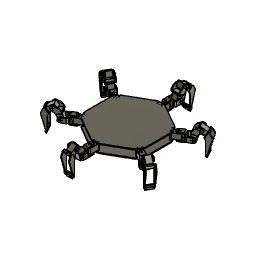
Final Iteration for VREP (Autodesk Fusion 360 design; units mm, degrees)
Autodesk Fusion 360 part; units mm, degrees
(part 1 of 2)
sketch "Sketch1" plane through (0, 0, 0) normal (0, 0, 1) x (1, 0, 0)
  line L0 (-115.223, -83.8445) -> (-15, -141.7083)
  circle A0 centre (-8, 136.7083) radius 1
  circle A1 centre (122.3929, -61.426) radius 1
  line L1 (0, 0) -> (-182.8649, -105.5771) construction
  circle A2 centre (0, 0) radius 142.5 construction
  circle A3 centre (-114.3929, -75.2824) radius 1
  line L2 (0, 0) -> (-200, 0) construction
  line L3 (-15, 141.7083) -> (15, 141.7083)
  line L4 (115.223, 83.8445) -> (15, 141.7083)
  line L5 (-15, -141.7083) -> (15, -141.7083)
  circle A4 centre (114.3929, 75.2824) radius 1
  circle A5 centre (122.3929, 61.426) radius 1
  circle A6 centre (-122.3929, -61.426) radius 1
  line L6 (0, 0) -> (0, 70) construction
  line L7 (-15, 141.7083) -> (-115.223, 83.8445)
  line L8 (-130.223, -57.8638) -> (-115.223, -83.8445)
  circle A7 centre (114.3929, -75.2824) radius 1
  line L9 (-130.223, 57.8638) -> (-130.223, -57.8638)
  line L10 (15, -141.7083) -> (115.223, -83.8445)
  line L11 (130.223, -57.8638) -> (130.223, 57.8638)
  line L12 (130.223, 57.8638) -> (115.223, 83.8445)
  circle A8 centre (-8, -136.7083) radius 1
  circle A9 centre (8, -136.7083) radius 1
  circle A10 centre (-114.3929, 75.2824) radius 1
  line L13 (130.223, -57.8638) -> (115.223, -83.8445)
  circle A11 centre (-122.3929, 61.426) radius 1
  line L14 (-130.223, 57.8638) -> (-115.223, 83.8445)
  line L15 (-128.4918, -62.4457) -> (-84.3692, -138.8683) construction
  circle A12 centre (8, 136.7083) radius 1
  dimension "d1" = 285
  dimension "d2" = 30
  dimension "d3" = 30
  dimension "d4" = 2
  dimension "d5" = 5
  dimension "d6" = 8
  dimension "d7" = 2
  dimension "d8" = 16
  dimension "d9" = 30
  dimension "d10" = 2
  dimension "d11" = 30
  dimension "d12" = 15
  dimension "d13" = 5
  dimension "d14" = 8
  dimension "d15" = 5
  constraint coincident L1.start A2.centre
  constraint coincident L0.end A2
  constraint coincident L5.end A2
  constraint horizontal L5
  constraint coincident L3.start A2
  constraint coincident L3.end A2
  constraint horizontal L3
  constraint parallel L2 L3
  constraint perpendicular L1 L15
  constraint tangent A2 L15
  constraint coincident L8.start A2
  constraint coincident L0.start A2
  constraint symmetric L1 A3 A6
  constraint symmetric A3 L2 A10
  constraint symmetric L8.start L9.start L2
  constraint symmetric L7.end L0.start L2
  constraint symmetric L2 A6 A11
  constraint perpendicular L2 L6
  constraint symmetric A3 L6 A7
  constraint symmetric L8.start L11.start L6
  constraint symmetric L10.end L0.start L6
  constraint symmetric A1 A6 L6
  constraint symmetric A5 L6 A11
  constraint symmetric A4 L6 A10
  constraint symmetric L11.end L9.start L6
  constraint symmetric L7.end L4.start L6
  constraint symmetric L2 A9 A12
  constraint symmetric A0 L2 A8
  measures "d1" diameter of A2
  measures "d2" distance of L5.end L0.end
  measures "d3" distance of L3.start L3.end
  measures "d4" diameter of A12
  measures "d5" distance of A12.centre L3
  measures "d6" horizontal distance of L1.start A12.centre
  measures "d7" diameter of A0
  measures "d8" horizontal distance of A12.centre A0.centre
  measures "d9" angle of L1 L2
  measures "d10" diameter of A3
  measures "d11" distance of L8.start L0.start
  measures "d12" distance of L0.start L1
  measures "d13" distance of A3.centre L8
  measures "d14" distance of A3.centre L1
  measures "d15" distance of A0.centre L3
extrude "Extrude1" add sketch "Sketch1" along normal blind 3.5 makes body 1
sketch "Sketch2" plane through (0, 0, 3.5) normal (0, 0, 1) x (-1, 0, 0)
  circle A0 centre (8, -136.7083) radius 1
  circle A1 centre (122.3929, 61.426) radius 1
  circle A2 centre (8, 136.7083) radius 1
  circle A3 centre (114.3929, -75.2824) radius 1
  circle A4 centre (-114.3929, 75.2824) radius 1
  circle A5 centre (-122.3929, 61.426) radius 1
  circle A6 centre (114.3929, 75.2824) radius 1
  circle A7 centre (-114.3929, -75.2824) radius 1
  circle A8 centre (-122.3929, -61.426) radius 1
  circle A9 centre (122.3929, -61.426) radius 1
  circle A10 centre (-8, -136.7083) radius 1
  circle A11 centre (-8, 136.7083) radius 1
  line L0 (130.223, 57.8638) -> (115.223, 83.8445)
  line L1 (115.223, 83.8445) -> (15, 141.7083)
  line L2 (15, 141.7083) -> (-15, 141.7083)
  line L3 (-15, 141.7083) -> (-115.223, 83.8445)
  line L4 (-115.223, 83.8445) -> (-130.223, 57.8638)
  line L5 (-130.223, 57.8638) -> (-130.223, -57.8638)
  line L6 (-130.223, -57.8638) -> (-115.223, -83.8445)
  line L7 (-115.223, -83.8445) -> (-15, -141.7083)
  line L8 (-15, -141.7083) -> (15, -141.7083)
  line L9 (15, -141.7083) -> (115.223, -83.8445)
  line L10 (115.223, -83.8445) -> (130.223, -57.8638)
  line L11 (130.223, -57.8638) -> (130.223, 57.8638)
  circle A12 centre (-122.3929, 61.426) radius 1
  circle A13 centre (-114.3929, 75.2824) radius 1
  circle A14 centre (-8, 136.7083) radius 1
  circle A15 centre (8, 136.7083) radius 1
  circle A16 centre (114.3929, 75.2824) radius 1
  circle A17 centre (122.3929, 61.426) radius 1
  line L12 (-115.223, 83.8445) -> (-130.223, 57.8638)
  line L13 (15, 141.7083) -> (-15, 141.7083)
  line L14 (130.223, 57.8638) -> (115.223, 83.8445)
  line L15 (115.223, 83.8445) -> (130.223, 57.8638)
  line L16 (-114.3929, 75.2824) -> (-110.0628, 72.7824) construction
  line L17 (-110.0628, 72.7824) -> (-108.5628, 75.3804) construction
  line L18 (-108.5628, 75.3804) -> (-112.8929, 77.8804)
  line L19 (-108.5628, 75.3804) -> (-108.6561, 75.2188)
  line L20 (-108.5628, 75.3804) -> (-119.5628, 56.3279)
  line L21 (-119.5628, 56.3279) -> (-123.8929, 58.8279)
  arc A18 (-112.8929, 77.8804) -> (-115.8929, 72.6843) centre (-114.3929, 75.2824) ccw
  arc A19 (-120.8929, 64.024) -> (-123.8929, 58.8279) centre (-122.3929, 61.426) ccw
  line L22 (-120.8929, 64.024) -> (-115.8929, 72.6843)
  line L23 (-108.5628, -75.3804) -> (-112.8929, -77.8804)
  arc A20 (-115.8929, -72.6843) -> (-112.8929, -77.8804) centre (-114.3929, -75.2824) ccw
  line L24 (-115.8929, -72.6843) -> (-120.8929, -64.024)
  arc A21 (-123.8929, -58.8279) -> (-120.8929, -64.024) centre (-122.3929, -61.426) ccw
  line L25 (-119.5628, -56.3279) -> (-123.8929, -58.8279)
  line L26 (-119.5628, -56.3279) -> (-108.5628, -75.3804)
  line L27 (11, -131.7083) -> (11, -136.7083)
  arc A22 (5, -136.7083) -> (11, -136.7083) centre (8, -136.7083) ccw
  line L28 (5, -136.7083) -> (-5, -136.7083)
  arc A23 (-11, -136.7083) -> (-5, -136.7083) centre (-8, -136.7083) ccw
  line L29 (-11, -131.7083) -> (-11, -136.7083)
  line L30 (-11, -131.7083) -> (11, -131.7083)
  line L31 (119.5628, -56.3279) -> (123.8929, -58.8279)
  arc A24 (120.8929, -64.024) -> (123.8929, -58.8279) centre (122.3929, -61.426) ccw
  line L32 (120.8929, -64.024) -> (115.8929, -72.6843)
  arc A25 (112.8929, -77.8804) -> (115.8929, -72.6843) centre (114.3929, -75.2824) ccw
  line L33 (108.5628, -75.3804) -> (112.8929, -77.8804)
  line L34 (108.5628, -75.3804) -> (119.5628, -56.3279)
  line L35 (108.5628, 75.3804) -> (112.8929, 77.8804)
  arc A26 (115.8929, 72.6843) -> (112.8929, 77.8804) centre (114.3929, 75.2824) ccw
  line L36 (115.8929, 72.6843) -> (120.8929, 64.024)
  arc A27 (123.8929, 58.8279) -> (120.8929, 64.024) centre (122.3929, 61.426) ccw
  line L37 (119.5628, 56.3279) -> (123.8929, 58.8279)
  line L38 (119.5628, 56.3279) -> (108.5628, 75.3804)
  line L39 (-11, 131.7083) -> (-11, 136.7083)
  arc A28 (-5, 136.7083) -> (-11, 136.7083) centre (-8, 136.7083) ccw
  line L40 (-5, 136.7083) -> (5, 136.7083)
  arc A29 (11, 136.7083) -> (5, 136.7083) centre (8, 136.7083) ccw
  line L41 (11, 131.7083) -> (11, 136.7083)
  line L42 (11, 131.7083) -> (-11, 131.7083)
  dimension "d22" = 6
  dimension "d23" = 6
  dimension "d24" = 5
  dimension "d25" = 90
  dimension "d27" = 22
  dimension "d29" = 360
  constraint concentric A12 A19
  constraint concentric A4 A18
  constraint coincident A4.centre A13.centre
  constraint perpendicular L12 L16
  constraint perpendicular L16 L17
  constraint perpendicular L12 L18
  constraint tangent L18 A18
  constraint coincident L17 L19.end
  constraint perpendicular L18 L20
  constraint perpendicular L20 L21
  measures "d22" diameter of A19
  measures "d23" diameter of A18
  measures "d24" distance of A4.centre L16.end
  measures "d25" angle of L12 L16
  measures "d27" distance of L17.end L20.end
extrude "Extrude2" add sketch "Sketch2" along normal blind 3.5 contours L18 L19 L20 L21 A18 A19 L22 | L23 A20 L24 A21 L25 L26 | L27 A22 L28 A23 L29 L30 | L31 A24 L32 A25 L33 L34 | L35 A26 L36 A27 L37 L38 | L39 A28 L40 A29 L41 L42 bodies 1
sketch "Sketch3" plane through (0, 0, 7) normal (0, 0, 1) x (-1, 0, 0)
  circle A0 centre (122.3929, 61.426) radius 1
  circle A1 centre (114.3929, 75.2824) radius 1
  arc A2 (123.8929, 58.8279) -> (120.8929, 64.024) centre (122.3929, 61.426) ccw
  line L0 (120.8929, 64.024) -> (115.8929, 72.6843)
  arc A3 (115.8929, 72.6843) -> (112.8929, 77.8804) centre (114.3929, 75.2824) ccw
  line L1 (112.8929, 77.8804) -> (108.5628, 75.3804)
  line L2 (108.5628, 75.3804) -> (119.5628, 56.3279)
  line L3 (119.5628, 56.3279) -> (123.8929, 58.8279)
  circle A4 centre (122.3929, -61.426) radius 1
  circle A5 centre (114.3929, -75.2824) radius 1
  line L4 (114.3929, -75.2824) -> (122.3929, -61.426) construction
  line L5 (122.3929, -61.426) -> (123.3929, -59.6939) construction
  line L6 (114.3929, -75.2824) -> (113.3929, -77.0144) construction
  line L7 (114.3929, -75.2824) -> (112.6608, -74.2824) construction
  line L8 (122.3929, -61.426) -> (120.6608, -60.426) construction
  line L9 (123.3929, -59.6939) -> (151.1057, -75.6939)
  line L10 (113.3929, -77.0144) -> (141.1057, -93.0144)
  line L11 (151.1057, -75.6939) -> (141.1057, -93.0144)
  line L12 (136.3833, -67.1939) -> (132.418, -74.062) construction
  circle A6 centre (148.3736, -76.426) radius 1
  circle A7 centre (140.3736, -90.2824) radius 1
  line L13 (123.8929, -58.8279) -> (119.5628, -56.3279)
  line L14 (119.5628, -56.3279) -> (108.5628, -75.3804)
  line L15 (108.5628, -75.3804) -> (112.8929, -77.8804)
  line L16 (113.3929, -77.0144) -> (112.8929, -77.8804)
  line L17 (123.3929, -59.6939) -> (123.8929, -58.8279)
  line L18 (123.3929, 59.6939) -> (151.1057, 75.6939)
  line L19 (141.1057, 93.0144) -> (151.1057, 75.6939)
  line L20 (113.3929, 77.0144) -> (141.1057, 93.0144)
  line L21 (113.3929, 77.0144) -> (112.8929, 77.8804)
  line L22 (112.8929, 77.8804) -> (108.5628, 75.3804)
  line L23 (108.5628, 75.3804) -> (119.5628, 56.3279)
  line L24 (119.5628, 56.3279) -> (123.8929, 58.8279)
  line L25 (123.3929, 59.6939) -> (123.8929, 58.8279)
  circle A8 centre (122.3929, 61.426) radius 1
  circle A9 centre (114.3929, 75.2824) radius 1
  circle A10 centre (140.3736, 90.2824) radius 1
  circle A11 centre (148.3736, 76.426) radius 1
  line L26 (10, 136.7083) -> (10, 168.7083)
  line L27 (-10, 168.7083) -> (10, 168.7083)
  line L28 (-10, 136.7083) -> (-10, 168.7083)
  line L29 (-10, 136.7083) -> (-11, 136.7083)
  line L30 (-11, 136.7083) -> (-11, 131.7083)
  line L31 (-11, 131.7083) -> (11, 131.7083)
  line L32 (11, 131.7083) -> (11, 136.7083)
  line L33 (10, 136.7083) -> (11, 136.7083)
  circle A12 centre (8, 136.7083) radius 1
  circle A13 centre (-8, 136.7083) radius 1
  circle A14 centre (-8, 166.7083) radius 1
  circle A15 centre (8, 166.7083) radius 1
  line L34 (-113.3929, 77.0144) -> (-141.1057, 93.0144)
  line L35 (-151.1057, 75.6939) -> (-141.1057, 93.0144)
  line L36 (-123.3929, 59.6939) -> (-151.1057, 75.6939)
  line L37 (-123.3929, 59.6939) -> (-123.8929, 58.8279)
  line L38 (-123.8929, 58.8279) -> (-119.5628, 56.3279)
  line L39 (-119.5628, 56.3279) -> (-108.5628, 75.3804)
  line L40 (-108.5628, 75.3804) -> (-112.8929, 77.8804)
  line L41 (-113.3929, 77.0144) -> (-112.8929, 77.8804)
  circle A16 centre (-114.3929, 75.2824) radius 1
  circle A17 centre (-122.3929, 61.426) radius 1
  circle A18 centre (-148.3736, 76.426) radius 1
  circle A19 centre (-140.3736, 90.2824) radius 1
  line L42 (-123.3929, -59.6939) -> (-151.1057, -75.6939)
  line L43 (-141.1057, -93.0144) -> (-151.1057, -75.6939)
  line L44 (-113.3929, -77.0144) -> (-141.1057, -93.0144)
  line L45 (-113.3929, -77.0144) -> (-112.8929, -77.8804)
  line L46 (-112.8929, -77.8804) -> (-108.5628, -75.3804)
  line L47 (-108.5628, -75.3804) -> (-119.5628, -56.3279)
  line L48 (-119.5628, -56.3279) -> (-123.8929, -58.8279)
  line L49 (-123.3929, -59.6939) -> (-123.8929, -58.8279)
  circle A20 centre (-122.3929, -61.426) radius 1
  circle A21 centre (-114.3929, -75.2824) radius 1
  circle A22 centre (-140.3736, -90.2824) radius 1
  circle A23 centre (-148.3736, -76.426) radius 1
  line L50 (-10, -136.7083) -> (-10, -168.7083)
  line L51 (10, -168.7083) -> (-10, -168.7083)
  line L52 (10, -136.7083) -> (10, -168.7083)
  line L53 (10, -136.7083) -> (11, -136.7083)
  line L54 (11, -136.7083) -> (11, -131.7083)
  line L55 (11, -131.7083) -> (-11, -131.7083)
  line L56 (-11, -131.7083) -> (-11, -136.7083)
  line L57 (-10, -136.7083) -> (-11, -136.7083)
  circle A24 centre (-8, -136.7083) radius 1
  circle A25 centre (8, -136.7083) radius 1
  circle A26 centre (8, -166.7083) radius 1
  circle A27 centre (-8, -166.7083) radius 1
  point P0 (122.3929, -61.426)
  point P1 (114.3929, -75.2824)
  dimension "d32" = 2
  dimension "d33" = 2
  dimension "d34" = 2
  dimension "d35" = 2
  dimension "d39" = 32
  dimension "d43" = 360
  constraint coincident P0 A4.centre
  constraint coincident P1 A5.centre
  constraint parallel L4 L5
  constraint parallel L4 L6
  constraint perpendicular L6 L7
  constraint perpendicular L4 L8
  constraint perpendicular L5 L9
  constraint perpendicular L6 L10
  constraint perpendicular L9 L12
  constraint symmetric A4 L12 A6
  constraint symmetric A5 L12 A7
  constraint coincident L15.end L16.end
  constraint coincident L13.start L17.end
  constraint coincident L9 L12.start
  measures "d32" distance of P0 L5.end
  measures "d33" distance of P1 L6.end
  measures "d34" distance of P1 L7.end
  measures "d35" distance of P0 L8.end
  measures "d39" distance of L6.end L10.end
extrude "Extrude3" add sketch "Sketch3" along normal blind 23 contours A2 L0 A3 L1 L2 L3 L18 L20 L21 L22 L23 L24 L25 | A2 L0 A3 L18 L19 L20 | L9 L10 L11 L13 L14 L15 L16 L17 | L26 L27 L28 L29 L30 L31 L32 L33 | L34 L35 L36 L37 L38 L39 L40 L41 | L42 L43 L44 L45 L46 L47 L48 L49 | L50 L51 L52 L53 L54 L55 L56 L57 bodies 1
sketch "Sketch5" plane through (0, 0, 30) normal (0, 0, 1) x (-1, 0, 0)
  circle A0 centre (8, 136.7083) radius 1
  circle A1 centre (8, 166.7083) radius 1
  circle A2 centre (-8, 166.7083) radius 1
  circle A3 centre (-8, 136.7083) radius 1
  line L0 (-10, 136.7083) -> (-11, 136.7083)
  line L1 (-11, 136.7083) -> (-11, 131.7083)
  line L2 (-11, 131.7083) -> (11, 131.7083)
  line L3 (11, 131.7083) -> (11, 136.7083)
  line L4 (11, 136.7083) -> (10, 136.7083)
  line L5 (10, 136.7083) -> (10, 168.7083)
  line L6 (10, 168.7083) -> (-10, 168.7083)
  line L7 (-10, 168.7083) -> (-10, 136.7083)
  line L8 (-123.8929, -58.8279) -> (-119.5628, -56.3279)
  line L9 (-119.5628, -56.3279) -> (-108.5628, -75.3804)
  line L10 (-108.5628, -75.3804) -> (-112.8929, -77.8804)
  arc A4 (-115.8929, -72.6843) -> (-112.8929, -77.8804) centre (-114.3929, -75.2824) ccw
  line L11 (-115.8929, -72.6843) -> (-120.8929, -64.024)
  arc A5 (-123.8929, -58.8279) -> (-120.8929, -64.024) centre (-122.3929, -61.426) ccw
  line L12 (11, 136.7083) -> (11, 131.7083)
  line L13 (11, 131.7083) -> (-11, 131.7083)
  line L14 (-11, 131.7083) -> (-11, 136.7083)
  arc A6 (-5, 136.7083) -> (-11, 136.7083) centre (-8, 136.7083) ccw
  line L15 (-5, 136.7083) -> (5, 136.7083)
  arc A7 (11, 136.7083) -> (5, 136.7083) centre (8, 136.7083) ccw
  line L16 (123.8929, 58.8279) -> (119.5628, 56.3279)
  line L17 (119.5628, 56.3279) -> (108.5628, 75.3804)
  line L18 (108.5628, 75.3804) -> (112.8929, 77.8804)
  arc A8 (115.8929, 72.6843) -> (112.8929, 77.8804) centre (114.3929, 75.2824) ccw
  line L19 (115.8929, 72.6843) -> (120.8929, 64.024)
  arc A9 (123.8929, 58.8279) -> (120.8929, 64.024) centre (122.3929, 61.426) ccw
  line L20 (-11, -136.7083) -> (-11, -131.7083)
  line L21 (-11, -131.7083) -> (11, -131.7083)
  line L22 (11, -131.7083) -> (11, -136.7083)
  arc A10 (5, -136.7083) -> (11, -136.7083) centre (8, -136.7083) ccw
  line L23 (5, -136.7083) -> (-5, -136.7083)
  arc A11 (-11, -136.7083) -> (-5, -136.7083) centre (-8, -136.7083) ccw
  line L24 (-108.5628, 75.3804) -> (-119.5628, 56.3279)
  line L25 (-119.5628, 56.3279) -> (-123.8929, 58.8279)
  arc A12 (-120.8929, 64.024) -> (-123.8929, 58.8279) centre (-122.3929, 61.426) ccw
  line L26 (-120.8929, 64.024) -> (-115.8929, 72.6843)
  arc A13 (-112.8929, 77.8804) -> (-115.8929, 72.6843) centre (-114.3929, 75.2824) ccw
  line L27 (-112.8929, 77.8804) -> (-108.5628, 75.3804)
  line L28 (112.8929, -77.8804) -> (108.5628, -75.3804)
  line L29 (108.5628, -75.3804) -> (119.5628, -56.3279)
  line L30 (119.5628, -56.3279) -> (123.8929, -58.8279)
  arc A14 (120.8929, -64.024) -> (123.8929, -58.8279) centre (122.3929, -61.426) ccw
  line L31 (120.8929, -64.024) -> (115.8929, -72.6843)
  arc A15 (112.8929, -77.8804) -> (115.8929, -72.6843) centre (114.3929, -75.2824) ccw
  line L32 (130.223, 57.8638) -> (115.223, 83.8445)
  line L33 (115.223, 83.8445) -> (15, 141.7083)
  line L34 (15, 141.7083) -> (-15, 141.7083)
  line L35 (-15, 141.7083) -> (-115.223, 83.8445)
  line L36 (-115.223, 83.8445) -> (-130.223, 57.8638)
  line L37 (-130.223, 57.8638) -> (-130.223, -57.8638)
  line L38 (-130.223, -57.8638) -> (-115.223, -83.8445)
  line L39 (-115.223, -83.8445) -> (-15, -141.7083)
  line L40 (-15, -141.7083) -> (15, -141.7083)
  line L41 (15, -141.7083) -> (115.223, -83.8445)
  line L42 (115.223, -83.8445) -> (130.223, -57.8638)
  line L43 (130.223, -57.8638) -> (130.223, 57.8638)
extrude "Extrude4" add sketch "Sketch5" along normal blind 3.5 contours L0 L1 L2 L3 L4 L5 L7 L12 L13 L14 A6 L15 A7 | L8 L9 L10 A4 L11 A5 | L16 L17 L18 A8 L19 A9 | L20 L21 L22 A10 L23 A11 | L24 L25 A12 L26 A13 L27 | L28 L29 L30 A14 L31 A15 bodies 1
sketch "Sketch6" plane through (0, 0, 33.5) normal (0, 0, 1) x (-1, 0, 0)
  line L0 (-119.5628, -56.3279) -> (-123.8929, -58.8279)
  arc A0 (-123.8929, -58.8279) -> (-120.8929, -64.024) centre (-122.3929, -61.426) ccw
  line L1 (-120.8929, -64.024) -> (-115.8929, -72.6843)
  arc A1 (-115.8929, -72.6843) -> (-112.8929, -77.8804) centre (-114.3929, -75.2824) ccw
  line L2 (-112.8929, -77.8804) -> (-108.5628, -75.3804)
  line L3 (-108.5628, -75.3804) -> (-119.5628, -56.3279)
  circle A2 centre (8, -136.7083) radius 1
  circle A3 centre (122.3929, 61.426) radius 1
  circle A4 centre (8, 136.7083) radius 1
  circle A5 centre (114.3929, -75.2824) radius 1
  circle A6 centre (-114.3929, 75.2824) radius 1
  circle A7 centre (-122.3929, 61.426) radius 1
  circle A8 centre (114.3929, 75.2824) radius 1
  circle A9 centre (-114.3929, -75.2824) radius 1
  circle A10 centre (-122.3929, -61.426) radius 1
  circle A11 centre (122.3929, -61.426) radius 1
  circle A12 centre (-8, -136.7083) radius 1
  circle A13 centre (-8, 136.7083) radius 1
  line L4 (115.223, 83.8445) -> (130.223, 57.8638)
  line L5 (130.223, 57.8638) -> (130.223, -57.8638)
  line L6 (130.223, -57.8638) -> (115.223, -83.8445)
  line L7 (115.223, -83.8445) -> (15, -141.7083)
  line L8 (15, -141.7083) -> (-15, -141.7083)
  line L9 (-15, -141.7083) -> (-115.223, -83.8445)
  line L10 (-115.223, -83.8445) -> (-130.223, -57.8638)
  line L11 (-130.223, -57.8638) -> (-130.223, 57.8638)
  line L12 (-130.223, 57.8638) -> (-115.223, 83.8445)
  line L13 (-115.223, 83.8445) -> (-15, 141.7083)
  line L14 (-15, 141.7083) -> (15, 141.7083)
  line L15 (15, 141.7083) -> (115.223, 83.8445)
extrude "Extrude5" add sketch "Sketch6" along normal blind 3.5 contours L0 A0 L1 A1 L2 L3 | L4 L5 L6 L7 L8 L9 L10 L11 L12 L13 L14 L15 bodies 1
sketch "Sketch7" plane through (0, 0, 30) normal (0, 0, 1) x (-1, 0, 0)
  arc A0 (125.3294, 60.8119) -> (120.8929, 64.024) centre (122.3929, 61.426) ccw
  line L0 (125.3294, 60.8119) -> (151.1057, 75.6939)
  line L1 (151.1057, 75.6939) -> (141.1057, 93.0144)
  line L2 (141.1057, 93.0144) -> (115.3294, 78.1325)
  arc A1 (115.8929, 72.6843) -> (115.3294, 78.1325) centre (114.3929, 75.2824) ccw
  line L3 (115.8929, 72.6843) -> (120.8929, 64.024)
  circle A2 centre (140.3736, 90.2824) radius 1
  circle A3 centre (148.3736, 76.426) radius 1
  line L4 (151.1057, 75.6939) -> (141.1057, 93.0144)
  line L5 (141.1057, 93.0144) -> (115.3294, 78.1325)
  line L6 (132.8785, 88.2644) -> (137.8785, 79.6042) construction
  line L7 (137.8785, 79.6042) -> (146.1057, 84.3542) construction
  circle A4 centre (137.8785, 79.6042) radius 7.8
  circle A5 centre (137.8785, 79.6042) radius 5.8 construction
  circle A6 centre (137.8785, 79.6042) radius 2.5
  line L8 (137.8785, 79.6042) -> (141.5223, 73.2929) construction
  line L9 (137.8785, 79.6042) -> (134.3704, 85.6803) construction
  line L10 (137.8785, 79.6042) -> (130.0691, 75.0954) construction
  circle A7 centre (142.9014, 82.5042) radius 1
  circle A8 centre (134.9628, 84.6542) radius 1
  circle A9 centre (132.8555, 76.7042) radius 1
  circle A10 centre (140.7785, 74.5812) radius 1
  circle A11 centre (-5.8313, 159.2083) radius 1
  circle A12 centre (0, 159.2083) radius 7.8
  circle A13 centre (0, 165.0083) radius 1
  circle A14 centre (5.8, 159.2083) radius 1
  circle A15 centre (0, 159.2083) radius 2.5
  circle A16 centre (0, 153.4083) radius 1
  circle A17 centre (-140.7941, 74.5541) radius 1
  circle A18 centre (-137.8785, 79.6042) radius 7.8
  circle A19 centre (-142.9014, 82.5042) radius 1
  circle A20 centre (-134.9785, 84.6271) radius 1
  circle A21 centre (-137.8785, 79.6042) radius 2.5
  circle A22 centre (-132.8555, 76.7042) radius 1
  circle A23 centre (-134.9628, -84.6542) radius 1
  circle A24 centre (-137.8785, -79.6042) radius 7.8
  circle A25 centre (-142.9014, -82.5042) radius 1
  circle A26 centre (-140.7785, -74.5812) radius 1
  circle A27 centre (-137.8785, -79.6042) radius 2.5
  circle A28 centre (-132.8555, -76.7042) radius 1
  circle A29 centre (5.8313, -159.2083) radius 1
  circle A30 centre (0, -159.2083) radius 7.8
  circle A31 centre (0, -165.0083) radius 1
  circle A32 centre (-5.8, -159.2083) radius 1
  circle A33 centre (0, -159.2083) radius 2.5
  circle A34 centre (0, -153.4083) radius 1
  circle A35 centre (140.7941, -74.5541) radius 1
  circle A36 centre (137.8785, -79.6042) radius 7.8
  circle A37 centre (142.9014, -82.5042) radius 1
  circle A38 centre (134.9785, -84.6271) radius 1
  circle A39 centre (137.8785, -79.6042) radius 2.5
  circle A40 centre (132.8555, -76.7042) radius 1
  dimension "d48" = 10
  dimension "d49" = 9.5
  dimension "d50" = 15.6
  dimension "d51" = 11.6
  dimension "d52" = 5
  dimension "d53" = 2
  dimension "d54" = 2
  dimension "d55" = 2
  dimension "d56" = 2
  dimension "d58" = 360
  constraint perpendicular L5 L6
  constraint midpoint L4 L7.end
  constraint coincident L6.end L7.start
  constraint concentric A4 A5
  constraint perpendicular L7 L8
  constraint coincident L6 L9.end
  constraint parallel L6 L9
  constraint perpendicular L9 L10
  constraint coincident A5 A7.centre
  constraint coincident L7 A7.centre
  constraint coincident L9 A8.centre
  constraint coincident A5 A9.centre
  constraint coincident L10 A9.centre
  constraint coincident A5 A10.centre
  constraint coincident L8 A10.centre
  measures "d48" distance of L6.start L6.end
  measures "d49" distance of L4 L6
  measures "d50" diameter of A4
  measures "d51" diameter of A5
  measures "d52" diameter of A6
  measures "d53" diameter of A7
  measures "d54" diameter of A8
  measures "d55" diameter of A9
  measures "d56" diameter of A10
extrude "Extrude6" add sketch "Sketch7" along normal blind 2.5 contours A4 | A12 | A18 | A24 | A30 | A36 bodies 1
sketch "Sketch8" plane through (0, 0, 7) normal (0, 0, -1) x (1, 0, 0)
  arc A0 (-125.3294, -60.8119) -> (-120.8929, -64.024) centre (-122.3929, -61.426) ccw
  line L0 (-125.3294, -60.8119) -> (-151.1057, -75.6939)
  line L1 (-151.1057, -75.6939) -> (-141.1057, -93.0144)
  line L2 (-141.1057, -93.0144) -> (-115.3294, -78.1325)
  arc A1 (-115.8929, -72.6843) -> (-115.3294, -78.1325) centre (-114.3929, -75.2824) ccw
  line L3 (-115.8929, -72.6843) -> (-120.8929, -64.024)
  circle A2 centre (-148.3736, -76.426) radius 1
  circle A3 centre (-140.3736, -90.2824) radius 1
  circle A4 centre (134.9785, 84.6271) radius 1
  circle A5 centre (137.8785, 79.6042) radius 2.5
  circle A6 centre (132.8555, 76.7042) radius 1
  circle A7 centre (140.7941, 74.5541) radius 1
  circle A8 centre (142.9014, 82.5042) radius 1
  circle A9 centre (137.8785, 79.6042) radius 7.8
  circle A10 centre (140.7785, -74.5812) radius 1
  circle A11 centre (132.8555, -76.7042) radius 1
  circle A12 centre (142.9014, -82.5042) radius 1
  circle A13 centre (137.8785, -79.6042) radius 2.5
  circle A14 centre (134.9628, -84.6542) radius 1
  circle A15 centre (137.8785, -79.6042) radius 7.8
  circle A16 centre (0, 153.4083) radius 1
  circle A17 centre (0, 159.2083) radius 2.5
  circle A18 centre (0, 165.0083) radius 1
  circle A19 centre (5.8313, 159.2083) radius 1
  circle A20 centre (-5.8, 159.2083) radius 1
  circle A21 centre (0, 159.2083) radius 7.8
  circle A22 centre (-137.8785, 79.6042) radius 2.5
  circle A23 centre (-140.7785, 74.5812) radius 1
  circle A24 centre (-142.9014, 82.5042) radius 1
  circle A25 centre (-134.9628, 84.6542) radius 1
  circle A26 centre (-132.8555, 76.7042) radius 1
  circle A27 centre (-137.8785, 79.6042) radius 7.8
  circle A28 centre (5.8, -159.2083) radius 1
  circle A29 centre (0, -159.2083) radius 2.5
  circle A30 centre (0, -165.0083) radius 1
  circle A31 centre (0, -153.4083) radius 1
  circle A32 centre (-5.8313, -159.2083) radius 1
  circle A33 centre (0, -159.2083) radius 7.8
  circle A34 centre (-134.9785, -84.6271) radius 1
  circle A35 centre (-140.7941, -74.5541) radius 1
  circle A36 centre (-142.9014, -82.5042) radius 1
  circle A37 centre (-137.8785, -79.6042) radius 2.5
  circle A38 centre (-132.8555, -76.7042) radius 1
  circle A39 centre (-137.8785, -79.6042) radius 7.8
extrude "Extrude7" add sketch "Sketch8" along normal blind 2.5 contours A9 | A15 | A21 | A27 | A33 | A39 bodies 1
sketch "Sketch9" plane through (0, 0, 0) normal (1, 0, 0) x (0, 1, 0)
  line L0 (-159.2083, 32.5) -> (-159.2083, 33) construction
  line L1 (-159.2083, 33) -> (-149.2083, 33)
  line L2 (-149.2083, 33) -> (-149.2083, 36.5)
  line L3 (-149.2083, 36.5) -> (-177.7083, 36.5)
  line L4 (-182.7083, 31.5) -> (-182.7083, 5.5)
  line L5 (-177.7083, 0.5) -> (-149.2083, 0.5)
  line L6 (-149.2083, 0.5) -> (-149.2083, 4)
  line L7 (-149.2083, 4) -> (-174.2083, 4)
  line L8 (-179.2083, 9) -> (-179.2083, 28)
  line L9 (-174.2083, 33) -> (-159.2083, 33)
  arc A0 (-182.7083, 5.5) -> (-177.7083, 0.5) centre (-177.7083, 5.5) ccw
  arc A1 (-179.2083, 9) -> (-174.2083, 4) centre (-174.2083, 9) ccw
  arc A2 (-174.2083, 33) -> (-179.2083, 28) centre (-174.2083, 28) ccw
  arc A3 (-177.7083, 36.5) -> (-182.7083, 31.5) centre (-177.7083, 31.5) ccw
  point P0 (-159.2083, 4.5)
  point P1 (-159.2083, 32.5)
  point P2 (-182.7083, 36.5)
  point P3 (-182.7083, 0.5)
  point P4 (-179.2083, 4)
  dimension "d63" = 0.5
  dimension "d64" = 10
  dimension "d65" = 3.5
  dimension "d66" = 33.5
  dimension "d67" = 36
  dimension "d68" = 33.5
  dimension "d69" = 3.5
  dimension "d70" = 30
  dimension "d77" = 5
  dimension "d78" = 5
  dimension "d79" = 5
  dimension "d80" = 5
  constraint coincident P1 L0.start
  constraint vertical L0
  constraint perpendicular L0 L1
  constraint perpendicular L1 L2
  constraint perpendicular L2 L3
  constraint perpendicular L3 L4
  constraint perpendicular L4 L5
  constraint perpendicular L5 L6
  constraint perpendicular L6 L7
  constraint perpendicular L7 L8
  constraint coincident P3 L5
  constraint coincident P3 L4
  constraint tangent L5 A0
  constraint tangent L4 A0
  constraint coincident P4 L7
  constraint coincident P4 L8
  constraint tangent L7 A1
  constraint tangent L8 A1
  constraint tangent L8 A2
  constraint tangent L9 A2
  constraint coincident P2 L4
  constraint coincident P2 L3
  constraint tangent L4 A3
  constraint tangent L3 A3
  measures "d63" distance of P1 L0.end
  measures "d64" distance of L0.end L1.end
  measures "d65" distance of L1.end L2.end
  measures "d66" distance of L2.end P2
  measures "d67" distance of P2 P3
  measures "d68" distance of P3 L5.end
  measures "d69" distance of L5.end L6.end
  measures "d70" distance of L6.end P4
  measures "d77" radius of A0
  measures "d78" radius of A1
  measures "d79" radius of A2
  measures "d80" radius of A3
extrude "Extrude8" add sketch "Sketch9" along normal mid plane 20 separate body makes body 2
sketch "Sketch10" plane through (0, 0, 36.5) normal (0, 0, 1) x (-1, 0, 0)
  line L0 (-10, 177.7083) -> (-10, 149.2083)
  line L1 (-10, 149.2083) -> (10, 149.2083)
  line L2 (10, 149.2083) -> (10, 177.7083)
  circle A0 centre (0, 165.0083) radius 1
  circle A1 centre (0, 159.2083) radius 2.5
  circle A2 centre (-5.8313, 159.2083) radius 1
  circle A3 centre (0, 153.4083) radius 1
  circle A4 centre (5.8, 159.2083) radius 1
  circle A5 centre (0, 159.2083) radius 7.8
  line L3 (-10, 149.2083) -> (-10, 177.7083)
  line L4 (10, 149.2083) -> (-10, 149.2083)
  line L5 (10, 177.7083) -> (10, 149.2083)
  arc A6 (-10, 159.2083) -> (10, 159.2083) centre (0, 159.2083) ccw
  line L6 (10, 177.7083) -> (-10, 177.7083)
  constraint concentric A1 A6
  constraint tangent L3 A6
  constraint coincident L2 A6.end
  constraint coincident L0 A6.start
extrude "Extrude9" cut sketch "Sketch10" against normal blind 3.5 contours L0 L1 L3 L4 A6 | L1 L2 L4 L5 A6 | A0 | A1 | A2 | A3 | A4 bodies 2
sketch "Sketch11" plane through (0, 0, 0.5) normal (0, 0, -1) x (1, 0, 0)
  line L0 (-10, 149.2083) -> (10, 149.2083)
  line L1 (10, 149.2083) -> (10, 177.7083)
  line L2 (-10, 177.7083) -> (-10, 149.2083)
  circle A0 centre (5.8313, 159.2083) radius 1
  circle A1 centre (0, 153.4083) radius 1
  circle A2 centre (-5.8, 159.2083) radius 1
  circle A3 centre (0, 159.2083) radius 2.5
  circle A4 centre (0, 165.0083) radius 1
  circle A5 centre (0, 159.2083) radius 7.8
  arc A6 (-10, 159.2083) -> (10, 159.2083) centre (0, 159.2083) ccw
  line L3 (10, 177.7083) -> (-10, 177.7083)
extrude "Extrude10" cut sketch "Sketch11" against normal blind 3.5 contours L0 L2 A6 | L0 L1 A6 | A0 | A1 | A2 | A3 | A4 bodies 2
ref_plane "WorkPlane1" through (0, 0, 18.5) normal (0, 0, 1) x (1, 0, 0)
sketch "Sketch12" plane through (0, 0, 18.5) normal (0, 0, 1) x (1, 0, 0)
  line L0 (-10, -182.7083) -> (10, -182.7083)
  line L1 (0, -182.7083) -> (13, -182.7083)
  line L2 (18, -187.7083) -> (18, -216.2083)
  line L3 (18, -216.2083) -> (14.5, -216.2083)
  line L4 (14.5, -216.2083) -> (14.5, -191.2083)
  line L5 (0, -182.7083) -> (-13, -182.7083)
  line L6 (-18, -187.7083) -> (-18, -216.2083)
  line L7 (-18, -216.2083) -> (-14.5, -216.2083)
  line L8 (-14.5, -216.2083) -> (-14.5, -191.2083)
  line L9 (-9.5, -186.2083) -> (9.5, -186.2083)
  arc A0 (-13, -182.7083) -> (-18, -187.7083) centre (-13, -187.7083) ccw
  arc A1 (-9.5, -186.2083) -> (-14.5, -191.2083) centre (-9.5, -191.2083) ccw
  arc A2 (18, -187.7083) -> (13, -182.7083) centre (13, -187.7083) ccw
  arc A3 (14.5, -191.2083) -> (9.5, -186.2083) centre (9.5, -191.2083) ccw
  point P0 (18, -182.7083)
  point P1 (14.5, -186.2083)
  point P2 (-18, -182.7083)
  point P3 (-14.5, -186.2083)
  dimension "d82" = 18
  dimension "d83" = 33.5
  dimension "d84" = 3.5
  dimension "d85" = 30
  dimension "d86" = 18
  dimension "d87" = 33.5
  dimension "d88" = 3.5
  dimension "d89" = 30
  dimension "d90" = 5
  dimension "d91" = 5
  dimension "d92" = 5
  dimension "d93" = 5
  constraint midpoint L0 L1.start
  constraint parallel L0 L1
  constraint perpendicular L1 L2
  constraint perpendicular L2 L3
  constraint perpendicular L3 L4
  constraint parallel L0 L5
  constraint perpendicular L5 L6
  constraint perpendicular L6 L7
  constraint perpendicular L7 L8
  constraint coincident P2 L5
  constraint coincident P2 L6
  constraint tangent L5 A0
  constraint tangent L6 A0
  constraint coincident P3 L9
  constraint coincident P3 L8
  constraint tangent L9 A1
  constraint tangent L8 A1
  constraint coincident P0 L1
  constraint coincident P0 L2
  constraint tangent L1 A2
  constraint tangent L2 A2
  constraint coincident P1 L9
  constraint coincident P1 L4
  constraint tangent L9 A3
  constraint tangent L4 A3
  measures "d82" distance of L1.start P0
  measures "d83" distance of P0 L2.end
  measures "d84" distance of L2.end L3.end
  measures "d85" distance of L3.end P1
  measures "d86" distance of L1.start P2
  measures "d87" distance of P2 L6.end
  measures "d88" distance of L6.end L7.end
  measures "d89" distance of L7.end P3
  measures "d90" radius of A0
  measures "d91" radius of A1
  measures "d92" radius of A2
  measures "d93" radius of A3
extrude "Extrude11" add sketch "Sketch12" along normal mid plane 20 bodies 2
sketch "Sketch13" plane through (-18, 0, 0) normal (-1, 0, 0) x (0, -1, 0)
  line L0 (216.2083, 8.5) -> (216.2083, 28.5)
  line L1 (216.2083, 28.5) -> (187.7083, 28.5)
  line L2 (187.7083, 28.5) -> (187.7083, 8.5)
  line L3 (187.7083, 8.5) -> (216.2083, 8.5)
  line L4 (187.7083, 28.5) -> (216.2083, 28.5)
  line L5 (216.2083, 8.5) -> (216.2083, 28.5)
  line L6 (216.2083, 8.5) -> (187.7083, 8.5)
  line L7 (216.2083, 18.5) -> (206.2083, 18.5)
  circle A0 centre (206.2083, 18.5) radius 2.5
  circle A1 centre (212.0083, 18.5) radius 1
  circle A2 centre (206.2083, 24.3) radius 1
  circle A3 centre (200.4083, 18.5) radius 1
  circle A4 centre (206.2083, 12.7) radius 1
  arc A5 (207.2046, 24.2138) -> (211.9221, 19.4963) centre (206.2083, 18.5) ccw construction
  arc A6 (206.2083, 8.5) -> (206.2083, 28.5) centre (206.2083, 18.5) ccw
  dimension "d96" = 10
  dimension "d97" = 20
  dimension "d98" = 2
  dimension "d99" = 2
  dimension "d100" = 2
  dimension "d101" = 2
  dimension "d102" = 5
  dimension "d103" = 11.6
  constraint midpoint L5 L7.start
  constraint perpendicular L5 L7
  constraint coincident L7.end A0.centre
  constraint concentric A0 A6
  constraint concentric A5 A6
  constraint coincident A1.centre A5
  constraint coincident L7 A1.centre
  constraint coincident A2.centre A5
  constraint coincident A3.centre A5
  constraint coincident A4.centre A5
  constraint coincident A1 A5.end
  constraint coincident A2 A5.start
  constraint coincident L1 A6.end
  constraint coincident L3 A6.start
  measures "d96" distance of L7.start L7.end
  measures "d97" diameter of A6
  measures "d98" diameter of A1
  measures "d99" diameter of A2
  measures "d100" diameter of A3
  measures "d101" diameter of A4
  measures "d102" diameter of A0
  measures "d103" diameter of A5
extrude "Extrude12" cut sketch "Sketch13" against normal up to surface (36 mm away) contours L0 L3 L5 L6 A6 | L0 L1 L4 L5 A6 | L7 A1 | L7 A1 | A0 | A2 | A3 | A4 bodies 2
ref_plane "WorkPlane2" through (11.5, -203.7083, 18.5) normal (-1, 0, 0) x (0, -1, 0)
sketch "Sketch28" plane through (11.5, 0, 0) normal (-1, 0, 0) x (0, -1, 0)
  line L0 (233.7083, 7.5) -> (228.7083, 7.5) construction
  line L1 (233.7083, 29.5) -> (233.7083, 7.5) construction
  line L2 (223, 29.5) -> (233.7083, 29.5) construction
  arc A0 (228.7083, 29.5) -> (226.4723, 28.5) centre (228.7083, 26.5) ccw construction
  line L3 (196.7083, 28.5) -> (226.4723, 28.5) construction
  line L4 (196.7083, 8.5) -> (196.7083, 28.5) construction
  line L5 (226.4723, 8.5) -> (196.7083, 8.5) construction
  arc A1 (226.4723, 8.5) -> (228.7083, 7.5) centre (228.7083, 10.5) ccw construction
  circle A2 centre (228.7083, 10.5) radius 1 construction
  circle A3 centre (228.7083, 26.5) radius 1 construction
  circle A4 centre (198.7083, 26.5) radius 1 construction
  circle A5 centre (198.7083, 10.5) radius 1 construction
  circle A6 centre (206.2083, 18.5) radius 2.5
  arc A7 (220.8136, 35.7428) -> (222.3248, 37.6705) centre (219.4139, 38.3963) ccw
  line L6 (223.5344, 42.522) -> (222.3248, 37.6705)
  line L7 (202.1879, 47.8443) -> (223.5344, 42.522)
  line L8 (200.9783, 42.9928) -> (202.1879, 47.8443)
  arc A8 (200.9783, 42.9928) -> (201.4077, 40.5812) centre (203.8892, 42.267) ccw
  line L9 (194.2071, 11.7014) -> (201.4077, 40.5812)
  line L10 (213.613, 6.863) -> (194.2071, 11.7014)
  line L11 (220.8136, 35.7428) -> (213.613, 6.863)
  circle A9 centre (212.1563, 9.2874) radius 1
  circle A10 centre (196.6315, 13.1582) radius 1
  circle A11 centre (203.8892, 42.267) radius 1
  circle A12 centre (219.4139, 38.3963) radius 1
  dimension "d223" = 2
  dimension "d224" = 2
  dimension "d225" = 2
  dimension "d226" = 2
  dimension "d227" = 2
  dimension "d228" = 2
  dimension "d229" = 2
  dimension "d230" = 2
  dimension "d231" = 2
  dimension "d232" = 2
  dimension "d233" = 6
  dimension "d234" = 5
  constraint horizontal L3
  constraint horizontal L5
  constraint vertical L4
  constraint concentric A1 A2
  constraint horizontal L2
  constraint perpendicular L1 L2
  constraint perpendicular L0 L1
  constraint tangent L0 A1
  constraint coincident A0.start L2
  measures "d223" distance of A4.centre L3
  measures "d224" diameter of A4
  measures "d225" distance of A4.centre L4
  measures "d226" diameter of A5
  measures "d227" distance of A5.centre L5
  measures "d228" distance of A5.centre L4
  measures "d229" diameter of A2
  measures "d230" distance of A1.centre L5
  measures "d231" distance of A0.centre L3
  measures "d232" diameter of A3
  measures "d233" diameter of A1
  measures "d234" distance of A0.centre L1
extrude "Extrude26" add sketch "Sketch28" along normal blind 23 separate body makes body 3
sketch "Sketch29" plane through (11.5, 0, 0) normal (1, 0, 0) x (0, 1, 0)
  circle A0 centre (-203.8892, 42.267) radius 1
  circle A1 centre (-219.4139, 38.3963) radius 1
  circle A2 centre (-206.2083, 18.5) radius 2.5
  circle A3 centre (-196.6315, 13.1582) radius 1
  circle A4 centre (-212.1563, 9.2874) radius 1
  arc A5 (-201.4077, 40.5812) -> (-200.9783, 42.9928) centre (-203.8892, 42.267) ccw
  line L0 (-200.9783, 42.9928) -> (-202.1879, 47.8443)
  line L1 (-202.1879, 47.8443) -> (-223.5344, 42.522)
  line L2 (-223.5344, 42.522) -> (-222.3248, 37.6705)
  arc A6 (-222.3248, 37.6705) -> (-220.8136, 35.7428) centre (-219.4139, 38.3963) ccw
  line L3 (-220.8136, 35.7428) -> (-213.613, 6.863)
  line L4 (-213.613, 6.863) -> (-194.2071, 11.7014)
  line L5 (-194.2071, 11.7014) -> (-201.4077, 40.5812)
  circle A7 centre (-206.2083, 18.5) radius 7.8
  circle A8 centre (-200.4083, 18.5) radius 1
  circle A9 centre (-206.2083, 24.3) radius 1
  circle A10 centre (-212.0083, 18.5) radius 1
  circle A11 centre (-206.2083, 12.7) radius 1
  dimension "d239" = 15.6
  constraint concentric A2 A7
  measures "d239" diameter of A7
extrude "Extrude27" add sketch "Sketch29" along normal blind 2.5 contours A7 bodies 3
sketch "Sketch30" plane through (-11.5, 0, 0) normal (-1, 0, 0) x (0, -1, 0)
  circle A0 centre (203.8892, 42.267) radius 1
  circle A1 centre (219.4139, 38.3963) radius 1
  circle A2 centre (206.2083, 18.5) radius 2.5
  circle A3 centre (196.6315, 13.1582) radius 1
  circle A4 centre (212.1563, 9.2874) radius 1
  arc A5 (200.9783, 42.9928) -> (201.4077, 40.5812) centre (203.8892, 42.267) ccw
  line L0 (201.4077, 40.5812) -> (194.2071, 11.7014)
  line L1 (194.2071, 11.7014) -> (213.613, 6.863)
  line L2 (213.613, 6.863) -> (220.8136, 35.7428)
  arc A6 (220.8136, 35.7428) -> (222.3248, 37.6705) centre (219.4139, 38.3963) ccw
  line L3 (222.3248, 37.6705) -> (223.5344, 42.522)
  line L4 (223.5344, 42.522) -> (202.1879, 47.8443)
  line L5 (202.1879, 47.8443) -> (200.9783, 42.9928)
  circle A7 centre (206.2083, 18.5) radius 7.8
  circle A8 centre (206.2083, 24.3) radius 1
  circle A9 centre (212.0083, 18.5) radius 1
  circle A10 centre (206.2083, 12.7) radius 1
  circle A11 centre (200.4083, 18.5) radius 1
extrude "Extrude28" add sketch "Sketch30" along normal blind 2.5 contours A7 bodies 3
ref_plane "WorkPlane7" through (-15, -208.8708, 27.3536) normal (-1, 0, 0) x (0, -1, 0)
sketch "Sketch32" plane through (-15, 0, 0) normal (-1, 0, 0) x (0, -1, 0)
  line L0 (222.3248, 37.6705) -> (223.5344, 42.522)
  line L1 (223.5344, 42.522) -> (202.1879, 47.8443)
  line L2 (202.1879, 47.8443) -> (200.9783, 42.9928)
  circle A0 centre (203.8892, 42.267) radius 1
  circle A1 centre (219.4139, 38.3963) radius 1
  line L3 (216.503, 39.122) -> (206.8001, 41.5413)
  arc A2 (216.503, 39.122) -> (222.3248, 37.6705) centre (219.4139, 38.3963) ccw
  arc A3 (200.9783, 42.9928) -> (206.8001, 41.5413) centre (203.8892, 42.267) ccw
  line L4 (206.8001, 41.5413) -> (216.503, 39.122)
  constraint concentric A1 A2
extrude "Extrude29" add sketch "Sketch32" against normal blind 30 bodies 3
sketch "Sketch33" plane through (-15, 0, 0) normal (-1, 0, 0) x (0, -1, 0)
  circle A0 centre (219.4139, 38.3963) radius 1
  circle A1 centre (203.8892, 42.267) radius 1
  line L0 (206.8001, 41.5413) -> (216.503, 39.122)
  arc A2 (216.503, 39.122) -> (222.3248, 37.6705) centre (219.4139, 38.3963) ccw
  line L1 (222.3248, 37.6705) -> (223.5344, 42.522)
  line L2 (223.5344, 42.522) -> (202.1879, 47.8443)
  line L3 (202.1879, 47.8443) -> (200.9783, 42.9928)
  arc A3 (200.9783, 42.9928) -> (206.8001, 41.5413) centre (203.8892, 42.267) ccw
  circle A4 centre (206.2083, 18.5) radius 2.5
  line L4 (226.0339, 66.7401) -> (218.0281, 63.5264)
  arc A5 (234.1738, 48.4871) -> (226.0339, 66.7401) centre (229.7591, 57.4598) ccw
  circle A6 centre (231.2107, 63.2816) radius 1
  circle A7 centre (223.9394, 58.9196) radius 1
  circle A8 centre (228.411, 51.6132) radius 1
  line L5 (226.0528, 44.4914) -> (234.1738, 48.4871)
  line L6 (202.1887, 47.8474) -> (200.9783, 42.9928)
  line L7 (222.287, 37.6799) -> (223.4546, 42.364)
  arc A9 (226.1347, 44.5317) -> (223.4546, 42.364) centre (229.5773, 37.5348) ccw
  arc A10 (218.0281, 63.5264) -> (202.1887, 47.8474) centre (228.7239, 36.881) ccw
  circle A11 centre (229.7591, 57.4598) radius 2.5
  circle A12 centre (235.5809, 56.0083) radius 1
  point P0 (206.2083, 18.5)
  point P1 (235.5809, 56.0083)
  dimension "d249" = 15.596
  dimension "d250" = 57.424
  dimension "d251" = 2
  dimension "d252" = 5
  constraint coincident P0 A4.centre
  constraint tangent L5 A9
  constraint coincident L5 A9.start
  constraint tangent L4 A10
  constraint concentric A5 A11
  constraint coincident P1 A12.centre
  measures "d249" diameter of A9
  measures "d250" diameter of A10
  measures "d251" diameter of A12
  measures "d252" diameter of A11
extrude "Extrude30" add sketch "Sketch33" along normal blind 3.5 contours L0 A2 L1 L2 L3 A3 L6 | L1 L2 L4 A5 L5 L6 A9 A10 bodies 3
sketch "Sketch34" plane through (15, 0, 0) normal (1, 0, 0) x (0, 1, 0)
  circle A0 centre (-219.4139, 38.3963) radius 1
  circle A1 centre (-203.8892, 42.267) radius 1
  line L0 (-216.503, 39.122) -> (-206.8001, 41.5413)
  arc A2 (-206.8001, 41.5413) -> (-200.9783, 42.9928) centre (-203.8892, 42.267) ccw
  line L1 (-200.9783, 42.9928) -> (-202.1879, 47.8443)
  line L2 (-202.1879, 47.8443) -> (-223.5344, 42.522)
  line L3 (-223.5344, 42.522) -> (-222.3248, 37.6705)
  arc A3 (-222.3248, 37.6705) -> (-216.503, 39.122) centre (-219.4139, 38.3963) ccw
  line L4 (-223.5344, 42.522) -> (-202.1879, 47.8443)
  line L5 (-202.1879, 47.8443) -> (-202.1887, 47.8474)
  arc A4 (-202.1887, 47.8474) -> (-218.0281, 63.5264) centre (-228.7239, 36.881) ccw
  line L6 (-218.0281, 63.5264) -> (-226.0339, 66.7401)
  arc A5 (-226.0339, 66.7401) -> (-234.1738, 48.4871) centre (-229.7591, 57.4598) ccw
  line L7 (-234.1738, 48.4871) -> (-226.1347, 44.5317)
  arc A6 (-223.5134, 42.4376) -> (-226.1347, 44.5317) centre (-229.5773, 37.5348) ccw
  line L8 (-223.5134, 42.4376) -> (-223.5344, 42.522)
  circle A7 centre (-229.7591, 57.4598) radius 2.5
  circle A8 centre (-231.2107, 63.2816) radius 1
  circle A9 centre (-223.9394, 58.9196) radius 1
  circle A10 centre (-228.411, 51.6132) radius 1
  circle A11 centre (-235.5809, 56.0083) radius 1
extrude "Extrude31" add sketch "Sketch34" along normal blind 3.5 bodies 3
ref_plane "WorkPlane8" through (14, -221.5333, 52.6811) normal (1, 0, 0) x (0, 1, 0)
sketch "Sketch35" plane through (14, 0, 0) normal (1, 0, 0) x (0, 1, 0)
  circle A0 centre (-231.2107, 63.2816) radius 1
  circle A1 centre (-223.9394, 58.9196) radius 1
  circle A2 centre (-229.7591, 57.4598) radius 2.5
  circle A3 centre (-235.5809, 56.0083) radius 1
  circle A4 centre (-228.411, 51.6132) radius 1
  circle A5 centre (-229.7591, 57.4598) radius 7.8
  circle A6 centre (-206.2083, 18.5) radius 2.5
  point P0 (-206.2083, 18.5)
  dimension "d258" = 15.6
  constraint concentric A2 A5
  constraint coincident P0 A6.centre
  measures "d258" diameter of A5
extrude "Extrude32" add sketch "Sketch35" against normal blind 28 separate body contours A5 makes body 4
ref_plane "WorkPlane9" through (11.5, -229.7591, 57.4598) normal (1, 0, 0) x (0, 1, 0)
sketch "Sketch36" plane through (11.5, 0, 0) normal (1, 0, 0) x (0, 1, 0)
  circle A0 centre (-206.2083, 18.5) radius 2.5
  circle A1 centre (-229.7591, 57.4598) radius 3.4
  line L0 (-227.0963, 70.9935) -> (-216.3797, 54.1069)
  line L1 (-216.3797, 54.1069) -> (-241.5103, 38.1586)
  line L2 (-242.8624, 36.1161) -> (-247.084, 33.437)
  line L3 (-247.084, 33.437) -> (-258.8722, 52.0122)
  line L4 (-258.8722, 52.0122) -> (-254.6506, 54.6913)
  arc A2 (-252.2268, 55.0451) -> (-254.6506, 54.6913) centre (-253.0431, 52.1583) ccw
  line L5 (-252.2268, 55.0451) -> (-227.0963, 70.9935)
  arc A3 (-242.8624, 36.1161) -> (-241.5103, 38.1586) centre (-244.4699, 38.6491) ccw
  circle A4 centre (-244.4699, 38.6491) radius 1
  circle A5 centre (-253.0431, 52.1583) radius 1
  point P0 (-206.2083, 18.5)
  constraint coincident P0 A0.centre
extrude "Extrude33" add sketch "Sketch36" against normal blind 23 contours L0 L1 L2 L3 L4 A2 L5 A3 bodies 4
ref_plane "WorkPlane10" through (-15, -237.626, 52.2152) normal (-1, 0, 0) x (0, -1, 0)
sketch "Sketch37" plane through (-15, 0, 0) normal (-1, 0, 0) x (0, -1, 0)
  circle A0 centre (253.0431, 52.1583) radius 1
  circle A1 centre (244.4699, 38.6491) radius 1
  line L0 (242.8624, 36.1161) -> (247.084, 33.437)
  line L1 (258.8722, 52.0122) -> (254.6506, 54.6913)
  arc A2 (254.6506, 54.6913) -> (251.4356, 49.6254) centre (253.0431, 52.1583) ccw
  line L2 (252.5073, 51.314) -> (253.0431, 52.1583)
  arc A3 (246.0774, 41.1821) -> (242.8624, 36.1161) centre (244.4699, 38.6491) ccw
  line L3 (244.4699, 38.6491) -> (245.0057, 39.4934)
  line L4 (246.0774, 41.1821) -> (251.4356, 49.6254)
  line L5 (258.8722, 52.0122) -> (247.084, 33.437)
  constraint concentric A0 A2
  constraint tangent L1 A2
  constraint concentric A1 A3
  constraint tangent L0 A3
  constraint coincident A1.centre A3.centre
  constraint coincident A0.centre A2.centre
  constraint coincident A0 L2.start
  constraint collinear L2 L3
  constraint coincident A3.start L3
  constraint coincident A1 L3.end
  constraint collinear L3 L4
  constraint perpendicular L0 L5
extrude "Extrude34" add sketch "Sketch37" against normal blind 30 bodies 4
sketch "Sketch38" plane through (0, 0, 0) normal (0, 0, 1) x (1, 0, 0)
sketch "Sketch39" plane through (-15, 0, 0) normal (-1, 0, 0) x (0, -1, 0)
  circle A0 centre (253.0431, 52.1583) radius 1
  circle A1 centre (244.4699, 38.6491) radius 1
  arc A2 (254.6506, 54.6913) -> (251.4356, 49.6254) centre (253.0431, 52.1583) ccw
  line L0 (251.4356, 49.6254) -> (246.0774, 41.1821)
  arc A3 (246.0774, 41.1821) -> (242.8624, 36.1161) centre (244.4699, 38.6491) ccw
  line L1 (242.8624, 36.1161) -> (247.084, 33.437)
  line L2 (247.084, 33.437) -> (258.8722, 52.0122)
  line L3 (258.8722, 52.0122) -> (254.6506, 54.6913)
  circle A4 centre (206.2083, 18.5) radius 2.5
  circle A5 centre (229.7591, 57.4598) radius 2.5
  line L4 (241.7002, 37.4962) -> (245.8335, 27.5664)
  line L5 (246.3282, 24.8623) -> (246.9237, -31.9835)
  arc A6 (246.3282, 24.8623) -> (245.7143, 27.8528) centre (238.3286, 24.7785) ccw
  line L6 (267.0495, 31.0174) -> (253.1035, -20.86)
  arc A7 (267.0495, 31.0174) -> (266.7096, 36.1683) centre (259.3238, 33.0942) ccw
  line L7 (261.5307, 48.6113) -> (266.7096, 36.1683)
  arc A8 (261.5307, 48.6113) -> (258.4315, 52.2919) centre (254.1449, 45.5373) ccw
  line L8 (253.2356, -31.3463) -> (252.8389, -23.3324)
  arc A9 (253.1035, -20.86) -> (252.8389, -23.3324) centre (260.8292, -22.9369) ccw
  arc A10 (251.6744, -33.3971) -> (253.2356, -31.3463) centre (251.2381, -31.4452) ccw
  line L9 (251.6744, -33.3971) -> (249.3599, -33.9144)
  arc A11 (246.9237, -31.9835) -> (249.3599, -33.9144) centre (248.9236, -31.9626) ccw
  circle A12 centre (249.9129, -30.9524) radius 1
  circle A13 centre (249.8605, -25.9531) radius 1
  point P0 (206.2083, 18.5)
  point P1 (229.7591, 57.4598)
  constraint coincident P0 A4.centre
  constraint coincident P1 A5.centre
extrude "Extrude35" add sketch "Sketch39" along normal blind 3.5 contours A2 L0 A3 L1 L2 L3 A8 | A3 L1 L2 L4 L5 A6 L6 A7 L7 A8 L8 A9 A10 L9 A11 bodies 4